Autodesk Fusion 360 part; units mm, degrees
(part 3 of 3)
  spline S39 degree 5 poles (-99.0173, 38.0348) (-99.0187, 38.0286) (-99.0216, 38.0164) (-99.0258, 37.9981) (-99.0314, 37.9737) (-99.0383, 37.9431) (-99.045, 37.9126) (-99.0515, 37.8821) (-99.058, 37.8516) (-99.0642, 37.8212) (-99.0704, 37.7907) (-99.0763, 37.7603) (-99.0822, 37.7298) (-99.0878, 37.6994) (-99.0934, 37.669) (-99.0987, 37.6387) (-99.104, 37.6083) (-99.1091, 37.578) (-99.114, 37.5477) (-99.1187, 37.5174) (-99.1234, 37.4871) (-99.1278, 37.4568) (-99.1321, 37.4266) (-99.1363, 37.3964) (-99.1403, 37.3662) (-99.1441, 37.3361) (-99.1478, 37.3059) (-99.1513, 37.2758) (-99.1546, 37.2457) (-99.1578, 37.2157) (-99.1608, 37.1857) (-99.1637, 37.1557) (-99.1663, 37.1257) (-99.1689, 37.0958) (-99.1712, 37.0659) (-99.1734, 37.036) (-99.1754, 37.0062) (-99.1772, 36.9764) (-99.1788, 36.9466) (-99.1803, 36.9169) (-99.1816, 36.8872) (-99.1827, 36.8576) (-99.1836, 36.8279) (-99.1843, 36.7984) (-99.1848, 36.7689) (-99.1851, 36.7394) (-99.1853, 36.7099) (-99.1852, 36.6805) (-99.185, 36.6512) (-99.1846, 36.6219) (-99.1839, 36.5926) (-99.183, 36.5634) (-99.1819, 36.5343) (-99.1805, 36.5052) (-99.179, 36.4762) (-99.1772, 36.4472) (-99.1752, 36.4183) (-99.173, 36.3895) (-99.1705, 36.3607) (-99.1679, 36.332) (-99.1649, 36.3033) (-99.1616, 36.2748) (-99.1579, 36.2463) (-99.1538, 36.218) (-99.1494, 36.1898) (-99.1448, 36.1616) (-99.1401, 36.1335) (-99.1351, 36.1054) (-99.1299, 36.0775) (-99.1242, 36.0497) (-99.1177, 36.0221) (-99.1117, 36.0003) (-99.1066, 35.9841) (-99.103, 35.9734) (-99.1011, 35.9681) knots -1 -1 -1 -1 -1 -1 -0.98571429 -0.97142857 -0.95714286 -0.94285714 -0.92857143 -0.91428571 -0.9 -0.88571429 -0.87142857 -0.85714286 -0.84285714 -0.82857143 -0.81428571 -0.8 -0.78571429 -0.77142857 -0.75714286 -0.74285714 -0.72857143 -0.71428571 -0.7 -0.68571429 -0.67142857 -0.65714286 -0.64285714 -0.62857143 -0.61428571 -0.6 -0.58571429 -0.57142857 -0.55714286 -0.54285714 -0.52857143 -0.51428571 -0.5 -0.48571429 -0.47142857 -0.45714286 -0.44285714 -0.42857143 -0.41428571 -0.4 -0.38571429 -0.37142857 -0.35714286 -0.34285714 -0.32857143 -0.31428571 -0.3 -0.28571429 -0.27142857 -0.25714286 -0.24285714 -0.22857143 -0.21428571 -0.2 -0.18571429 -0.17142857 -0.15714286 -0.14285714 -0.12857143 -0.11428571 -0.1 -0.08571429 -0.07142857 -0.05714286 -0.04285714 -0.02857143 -0.01428571 0 0 0 0 0 0
  line L39 (-99.1011, 35.9681) -> (-98.9382, 35.5089)
  arc A79 (-98.9981, 35.3816) -> (-98.9382, 35.5089) centre (-99.0325, 35.4755) ccw
  arc A80 (-98.9981, 35.3816) -> (-99.9434, 34.99) centre (-94.8448, 24.0176) ccw
  arc A81 (-100.0758, 35.0377) -> (-99.9434, 34.99) centre (-99.9856, 35.0807) ccw
  line L40 (-100.0758, 35.0377) -> (-100.2854, 35.4776)
  spline S40 degree 5 poles (-100.2854, 35.4776) (-100.2878, 35.4827) (-100.2928, 35.4928) (-100.3006, 35.5078) (-100.3118, 35.5275) (-100.3267, 35.5516) (-100.3423, 35.5753) (-100.3584, 35.5987) (-100.3747, 35.6221) (-100.3912, 35.6453) (-100.4079, 35.6685) (-100.4248, 35.6916) (-100.4419, 35.7145) (-100.4594, 35.7372) (-100.4773, 35.7597) (-100.4954, 35.7821) (-100.5138, 35.8043) (-100.5325, 35.8263) (-100.5513, 35.8483) (-100.5703, 35.8702) (-100.5896, 35.8919) (-100.609, 35.9135) (-100.6286, 35.9351) (-100.6484, 35.9565) (-100.6684, 35.9777) (-100.6886, 35.9989) (-100.709, 36.0199) (-100.7296, 36.0408) (-100.7504, 36.0617) (-100.7713, 36.0824) (-100.7924, 36.103) (-100.8136, 36.1235) (-100.835, 36.1439) (-100.8566, 36.1642) (-100.8783, 36.1844) (-100.9002, 36.2045) (-100.9223, 36.2245) (-100.9445, 36.2443) (-100.9669, 36.2641) (-100.9894, 36.2838) (-101.012, 36.3034) (-101.0348, 36.3229) (-101.0578, 36.3423) (-101.0808, 36.3616) (-101.1041, 36.3808) (-101.1274, 36.3999) (-101.1509, 36.4189) (-101.1746, 36.4378) (-101.1983, 36.4566) (-101.2222, 36.4753) (-101.2463, 36.4939) (-101.2704, 36.5124) (-101.2947, 36.5308) (-101.3191, 36.5492) (-101.3437, 36.5674) (-101.3683, 36.5855) (-101.3931, 36.6036) (-101.4181, 36.6215) (-101.4431, 36.6394) (-101.4683, 36.6572) (-101.4935, 36.6748) (-101.5189, 36.6924) (-101.5445, 36.7099) (-101.5701, 36.7273) (-101.5958, 36.7446) (-101.6217, 36.7618) (-101.6477, 36.7789) (-101.6738, 36.7959) (-101.7, 36.8129) (-101.7263, 36.8297) (-101.7527, 36.8465) (-101.774, 36.8598) (-101.7899, 36.8697) (-101.8006, 36.8763) (-101.806, 36.8797) knots 0 0 0 0 0 0 0.01428571 0.02857143 0.04285714 0.05714286 0.07142857 0.08571429 0.1 0.11428571 0.12857143 0.14285714 0.15714286 0.17142857 0.18571429 0.2 0.21428571 0.22857143 0.24285714 0.25714286 0.27142857 0.28571429 0.3 0.31428571 0.32857143 0.34285714 0.35714286 0.37142857 0.38571429 0.4 0.41428571 0.42857143 0.44285714 0.45714286 0.47142857 0.48571429 0.5 0.51428571 0.52857143 0.54285714 0.55714286 0.57142857 0.58571429 0.6 0.61428571 0.62857143 0.64285714 0.65714286 0.67142857 0.68571429 0.7 0.71428571 0.72857143 0.74285714 0.75714286 0.77142857 0.78571429 0.8 0.81428571 0.82857143 0.84285714 0.85714286 0.87142857 0.88571429 0.9 0.91428571 0.92857143 0.94285714 0.95714286 0.97142857 0.98571429 1 1 1 1 1 1
  arc A82 (-101.806, 36.8797) -> (-102.503, 36.4772) centre (-94.8448, 24.0176) ccw
  spline S41 degree 5 poles (-102.503, 36.4772) (-102.5028, 36.4709) (-102.5024, 36.4584) (-102.5018, 36.4396) (-102.5009, 36.4145) (-102.4996, 36.3833) (-102.4982, 36.3521) (-102.4966, 36.3209) (-102.4949, 36.2898) (-102.4931, 36.2587) (-102.4911, 36.2277) (-102.489, 36.1968) (-102.4868, 36.1659) (-102.4844, 36.135) (-102.4818, 36.1042) (-102.4792, 36.0735) (-102.4764, 36.0428) (-102.4734, 36.0122) (-102.4703, 35.9817) (-102.4671, 35.9512) (-102.4637, 35.9207) (-102.4602, 35.8904) (-102.4565, 35.86) (-102.4527, 35.8298) (-102.4488, 35.7996) (-102.4447, 35.7695) (-102.4404, 35.7394) (-102.436, 35.7095) (-102.4315, 35.6795) (-102.4268, 35.6497) (-102.4219, 35.6199) (-102.4169, 35.5902) (-102.4117, 35.5606) (-102.4064, 35.531) (-102.4009, 35.5015) (-102.3953, 35.4721) (-102.3895, 35.4428) (-102.3835, 35.4135) (-102.3774, 35.3843) (-102.3711, 35.3552) (-102.3647, 35.3262) (-102.3581, 35.2973) (-102.3513, 35.2685) (-102.3443, 35.2397) (-102.3372, 35.2111) (-102.3299, 35.1825) (-102.3224, 35.154) (-102.3148, 35.1256) (-102.3069, 35.0974) (-102.2989, 35.0692) (-102.2907, 35.0411) (-102.2823, 35.0131) (-102.2737, 34.9853) (-102.2648, 34.9575) (-102.2558, 34.9299) (-102.2466, 34.9024) (-102.2372, 34.875) (-102.2276, 34.8477) (-102.2178, 34.8205) (-102.2077, 34.7935) (-102.1975, 34.7666) (-102.1869, 34.7398) (-102.1759, 34.7133) (-102.1647, 34.687) (-102.1532, 34.6609) (-102.1414, 34.6349) (-102.1295, 34.6089) (-102.1175, 34.5831) (-102.1052, 34.5575) (-102.0925, 34.5321) (-102.0791, 34.5072) (-102.0676, 34.4877) (-102.0586, 34.4733) (-102.0523, 34.464) (-102.0491, 34.4593) knots -1 -1 -1 -1 -1 -1 -0.98571429 -0.97142857 -0.95714286 -0.94285714 -0.92857143 -0.91428571 -0.9 -0.88571429 -0.87142857 -0.85714286 -0.84285714 -0.82857143 -0.81428571 -0.8 -0.78571429 -0.77142857 -0.75714286 -0.74285714 -0.72857143 -0.71428571 -0.7 -0.68571429 -0.67142857 -0.65714286 -0.64285714 -0.62857143 -0.61428571 -0.6 -0.58571429 -0.57142857 -0.55714286 -0.54285714 -0.52857143 -0.51428571 -0.5 -0.48571429 -0.47142857 -0.45714286 -0.44285714 -0.42857143 -0.41428571 -0.4 -0.38571429 -0.37142857 -0.35714286 -0.34285714 -0.32857143 -0.31428571 -0.3 -0.28571429 -0.27142857 -0.25714286 -0.24285714 -0.22857143 -0.21428571 -0.2 -0.18571429 -0.17142857 -0.15714286 -0.14285714 -0.12857143 -0.11428571 -0.1 -0.08571429 -0.07142857 -0.05714286 -0.04285714 -0.02857143 -0.01428571 0 0 0 0 0 0
  line L41 (-102.0491, 34.4593) -> (-101.7729, 34.0579)
  arc A83 (-101.7978, 33.9194) -> (-101.7729, 34.0579) centre (-101.8553, 34.0012) ccw
  arc A84 (-101.7978, 33.9194) -> (-102.6096, 33.2965) centre (-94.8448, 24.0176) ccw
  arc A85 (-102.7498, 33.3083) -> (-102.6096, 33.2965) centre (-102.6737, 33.3732) ccw
  line L42 (-102.7498, 33.3083) -> (-103.066, 33.6789)
  spline S42 degree 5 poles (-103.066, 33.6789) (-103.0697, 33.6832) (-103.0772, 33.6917) (-103.0886, 33.7042) (-103.1045, 33.7203) (-103.1251, 33.7397) (-103.1464, 33.7586) (-103.168, 33.7771) (-103.1898, 33.7954) (-103.2117, 33.8136) (-103.2338, 33.8317) (-103.2561, 33.8496) (-103.2786, 33.8672) (-103.3014, 33.8847) (-103.3244, 33.9018) (-103.3477, 33.9187) (-103.3713, 33.9354) (-103.395, 33.9519) (-103.4189, 33.9682) (-103.4429, 33.9844) (-103.4671, 34.0004) (-103.4914, 34.0163) (-103.516, 34.032) (-103.5406, 34.0476) (-103.5655, 34.0629) (-103.5905, 34.0781) (-103.6156, 34.0932) (-103.6409, 34.108) (-103.6664, 34.1228) (-103.6919, 34.1374) (-103.7176, 34.1518) (-103.7435, 34.1661) (-103.7694, 34.1803) (-103.7955, 34.1943) (-103.8217, 34.2082) (-103.8481, 34.2219) (-103.8746, 34.2355) (-103.9012, 34.249) (-103.9279, 34.2623) (-103.9547, 34.2755) (-103.9817, 34.2886) (-104.0087, 34.3015) (-104.0359, 34.3143) (-104.0632, 34.3269) (-104.0906, 34.3395) (-104.1181, 34.3519) (-104.1457, 34.3641) (-104.1734, 34.3763) (-104.2013, 34.3883) (-104.2292, 34.4002) (-104.2572, 34.4119) (-104.2854, 34.4236) (-104.3136, 34.4351) (-104.3419, 34.4465) (-104.3704, 34.4577) (-104.3989, 34.4689) (-104.4275, 34.4799) (-104.4562, 34.4908) (-104.485, 34.5015) (-104.5139, 34.5122) (-104.5429, 34.5227) (-104.572, 34.5331) (-104.6012, 34.5434) (-104.6304, 34.5536) (-104.6598, 34.5636) (-104.6892, 34.5736) (-104.7188, 34.5834) (-104.7484, 34.5931) (-104.7781, 34.6026) (-104.8078, 34.6121) (-104.8377, 34.6214) (-104.8617, 34.6288) (-104.8797, 34.6343) (-104.8917, 34.6379) (-104.8977, 34.6397) knots 0 0 0 0 0 0 0.01428571 0.02857143 0.04285714 0.05714286 0.07142857 0.08571429 0.1 0.11428571 0.12857143 0.14285714 0.15714286 0.17142857 0.18571429 0.2 0.21428571 0.22857143 0.24285714 0.25714286 0.27142857 0.28571429 0.3 0.31428571 0.32857143 0.34285714 0.35714286 0.37142857 0.38571429 0.4 0.41428571 0.42857143 0.44285714 0.45714286 0.47142857 0.48571429 0.5 0.51428571 0.52857143 0.54285714 0.55714286 0.57142857 0.58571429 0.6 0.61428571 0.62857143 0.64285714 0.65714286 0.67142857 0.68571429 0.7 0.71428571 0.72857143 0.74285714 0.75714286 0.77142857 0.78571429 0.8 0.81428571 0.82857143 0.84285714 0.85714286 0.87142857 0.88571429 0.9 0.91428571 0.92857143 0.94285714 0.95714286 0.97142857 0.98571429 1 1 1 1 1 1
  arc A86 (-104.8977, 34.6397) -> (-105.4668, 34.0706) centre (-94.8448, 24.0176) ccw
  spline S43 degree 5 poles (-105.4668, 34.0706) (-105.465, 34.0645) (-105.4614, 34.0525) (-105.4559, 34.0345) (-105.4486, 34.0106) (-105.4392, 33.9807) (-105.4298, 33.9509) (-105.4202, 33.9212) (-105.4105, 33.8916) (-105.4007, 33.8621) (-105.3908, 33.8327) (-105.3807, 33.8033) (-105.3706, 33.774) (-105.3603, 33.7449) (-105.3499, 33.7158) (-105.3393, 33.6868) (-105.3287, 33.6579) (-105.3179, 33.6291) (-105.307, 33.6004) (-105.296, 33.5717) (-105.2849, 33.5432) (-105.2736, 33.5148) (-105.2622, 33.4865) (-105.2507, 33.4582) (-105.2391, 33.4301) (-105.2273, 33.4021) (-105.2154, 33.3741) (-105.2034, 33.3463) (-105.1913, 33.3186) (-105.179, 33.291) (-105.1666, 33.2635) (-105.1541, 33.2361) (-105.1414, 33.2088) (-105.1286, 33.1816) (-105.1157, 33.1545) (-105.1027, 33.1276) (-105.0895, 33.1007) (-105.0761, 33.074) (-105.0627, 33.0474) (-105.0491, 33.021) (-105.0353, 32.9946) (-105.0215, 32.9684) (-105.0075, 32.9423) (-104.9933, 32.9163) (-104.979, 32.8905) (-104.9645, 32.8648) (-104.9499, 32.8392) (-104.9352, 32.8138) (-104.9203, 32.7885) (-104.9053, 32.7633) (-104.8901, 32.7383) (-104.8747, 32.7135) (-104.8592, 32.6888) (-104.8435, 32.6643) (-104.8276, 32.64) (-104.8116, 32.6158) (-104.7954, 32.5917) (-104.779, 32.5679) (-104.7625, 32.5441) (-104.7459, 32.5206) (-104.729, 32.4973) (-104.7118, 32.4742) (-104.6944, 32.4514) (-104.6767, 32.4289) (-104.6588, 32.4067) (-104.6407, 32.3846) (-104.6225, 32.3626) (-104.6042, 32.3408) (-104.5857, 32.3192) (-104.5669, 32.298) (-104.5475, 32.2774) (-104.5314, 32.2615) (-104.5189, 32.25) (-104.5104, 32.2426) (-104.5061, 32.2389) knots -1 -1 -1 -1 -1 -1 -0.98571429 -0.97142857 -0.95714286 -0.94285714 -0.92857143 -0.91428571 -0.9 -0.88571429 -0.87142857 -0.85714286 -0.84285714 -0.82857143 -0.81428571 -0.8 -0.78571429 -0.77142857 -0.75714286 -0.74285714 -0.72857143 -0.71428571 -0.7 -0.68571429 -0.67142857 -0.65714286 -0.64285714 -0.62857143 -0.61428571 -0.6 -0.58571429 -0.57142857 -0.55714286 -0.54285714 -0.52857143 -0.51428571 -0.5 -0.48571429 -0.47142857 -0.45714286 -0.44285714 -0.42857143 -0.41428571 -0.4 -0.38571429 -0.37142857 -0.35714286 -0.34285714 -0.32857143 -0.31428571 -0.3 -0.28571429 -0.27142857 -0.25714286 -0.24285714 -0.22857143 -0.21428571 -0.2 -0.18571429 -0.17142857 -0.15714286 -0.14285714 -0.12857143 -0.11428571 -0.1 -0.08571429 -0.07142857 -0.05714286 -0.04285714 -0.02857143 -0.01428571 0 0 0 0 0 0
  line L43 (-104.5061, 32.2389) -> (-104.1355, 31.9227)
  arc A87 (-104.1237, 31.7824) -> (-104.1355, 31.9227) centre (-104.2004, 31.8466) ccw
  arc A88 (-104.1237, 31.7824) -> (-104.7465, 30.9707) centre (-94.8448, 24.0176) ccw
  arc A89 (-104.8851, 30.9458) -> (-104.7465, 30.9707) centre (-104.8284, 31.0281) ccw
  line L44 (-104.8851, 30.9458) -> (-105.2864, 31.2219)
  spline S44 degree 5 poles (-105.2864, 31.2219) (-105.2911, 31.2251) (-105.3005, 31.2314) (-105.3148, 31.2405) (-105.3343, 31.2519) (-105.3593, 31.2653) (-105.3846, 31.278) (-105.4103, 31.2903) (-105.4361, 31.3024) (-105.462, 31.3143) (-105.488, 31.326) (-105.5142, 31.3375) (-105.5405, 31.3488) (-105.567, 31.3597) (-105.5937, 31.3703) (-105.6206, 31.3806) (-105.6477, 31.3906) (-105.6748, 31.4004) (-105.7021, 31.41) (-105.7295, 31.4194) (-105.7571, 31.4287) (-105.7847, 31.4377) (-105.8124, 31.4465) (-105.8403, 31.4551) (-105.8682, 31.4636) (-105.8963, 31.4718) (-105.9245, 31.4798) (-105.9528, 31.4876) (-105.9812, 31.4953) (-106.0097, 31.5027) (-106.0382, 31.51) (-106.0669, 31.5172) (-106.0956, 31.5241) (-106.1245, 31.5309) (-106.1534, 31.5375) (-106.1824, 31.544) (-106.2115, 31.5503) (-106.2407, 31.5564) (-106.2699, 31.5623) (-106.2993, 31.5681) (-106.3287, 31.5738) (-106.3581, 31.5793) (-106.3877, 31.5846) (-106.4173, 31.5897) (-106.4471, 31.5948) (-106.4768, 31.5996) (-106.5067, 31.6043) (-106.5366, 31.6089) (-106.5666, 31.6133) (-106.5966, 31.6175) (-106.6268, 31.6216) (-106.6569, 31.6256) (-106.6872, 31.6294) (-106.7175, 31.6331) (-106.7479, 31.6366) (-106.7783, 31.64) (-106.8088, 31.6432) (-106.8394, 31.6463) (-106.87, 31.6492) (-106.9007, 31.652) (-106.9314, 31.6547) (-106.9622, 31.6572) (-106.993, 31.6596) (-107.0239, 31.6619) (-107.0549, 31.664) (-107.0859, 31.6659) (-107.1169, 31.6678) (-107.148, 31.6695) (-107.1792, 31.671) (-107.2104, 31.6724) (-107.2417, 31.6737) (-107.2667, 31.6746) (-107.2855, 31.6753) (-107.2981, 31.6757) (-107.3044, 31.6759) knots 0 0 0 0 0 0 0.01428571 0.02857143 0.04285714 0.05714286 0.07142857 0.08571429 0.1 0.11428571 0.12857143 0.14285714 0.15714286 0.17142857 0.18571429 0.2 0.21428571 0.22857143 0.24285714 0.25714286 0.27142857 0.28571429 0.3 0.31428571 0.32857143 0.34285714 0.35714286 0.37142857 0.38571429 0.4 0.41428571 0.42857143 0.44285714 0.45714286 0.47142857 0.48571429 0.5 0.51428571 0.52857143 0.54285714 0.55714286 0.57142857 0.58571429 0.6 0.61428571 0.62857143 0.64285714 0.65714286 0.67142857 0.68571429 0.7 0.71428571 0.72857143 0.74285714 0.75714286 0.77142857 0.78571429 0.8 0.81428571 0.82857143 0.84285714 0.85714286 0.87142857 0.88571429 0.9 0.91428571 0.92857143 0.94285714 0.95714286 0.97142857 0.98571429 1 1 1 1 1 1
  arc A90 (-107.3044, 31.6759) -> (-107.7068, 30.9788) centre (-94.8448, 24.0176) ccw
  spline S45 degree 5 poles (-107.7068, 30.9788) (-107.7035, 30.9735) (-107.6969, 30.9628) (-107.6869, 30.9468) (-107.6736, 30.9256) (-107.6569, 30.8992) (-107.64, 30.8728) (-107.6231, 30.8466) (-107.6061, 30.8205) (-107.589, 30.7946) (-107.5718, 30.7687) (-107.5544, 30.7429) (-107.5371, 30.7173) (-107.5196, 30.6918) (-107.502, 30.6664) (-107.4843, 30.6411) (-107.4666, 30.616) (-107.4487, 30.5909) (-107.4307, 30.566) (-107.4127, 30.5412) (-107.3945, 30.5165) (-107.3763, 30.492) (-107.358, 30.4676) (-107.3396, 30.4433) (-107.321, 30.4191) (-107.3024, 30.3951) (-107.2837, 30.3712) (-107.2649, 30.3474) (-107.246, 30.3238) (-107.227, 30.3003) (-107.2079, 30.2769) (-107.1887, 30.2537) (-107.1694, 30.2306) (-107.15, 30.2077) (-107.1305, 30.1849) (-107.111, 30.1622) (-107.0913, 30.1397) (-107.0715, 30.1174) (-107.0516, 30.0952) (-107.0316, 30.0731) (-107.0115, 30.0512) (-106.9913, 30.0295) (-106.971, 30.0079) (-106.9506, 29.9865) (-106.9301, 29.9652) (-106.9095, 29.9441) (-106.8888, 29.9232) (-106.868, 29.9025) (-106.8471, 29.8819) (-106.826, 29.8615) (-106.8049, 29.8412) (-106.7836, 29.8212) (-106.7622, 29.8014) (-106.7407, 29.7818) (-106.7191, 29.7624) (-106.6973, 29.7432) (-106.6755, 29.7242) (-106.6535, 29.7053) (-106.6314, 29.6867) (-106.6092, 29.6683) (-106.5869, 29.6501) (-106.5643, 29.6323) (-106.5416, 29.6148) (-106.5187, 29.5976) (-106.4956, 29.5807) (-106.4725, 29.5641) (-106.4492, 29.5476) (-106.4259, 29.5313) (-106.4024, 29.5152) (-106.3787, 29.4996) (-106.3546, 29.4847) (-106.335, 29.4735) (-106.32, 29.4656) (-106.3098, 29.4607) (-106.3047, 29.4582) knots -1 -1 -1 -1 -1 -1 -0.98571429 -0.97142857 -0.95714286 -0.94285714 -0.92857143 -0.91428571 -0.9 -0.88571429 -0.87142857 -0.85714286 -0.84285714 -0.82857143 -0.81428571 -0.8 -0.78571429 -0.77142857 -0.75714286 -0.74285714 -0.72857143 -0.71428571 -0.7 -0.68571429 -0.67142857 -0.65714286 -0.64285714 -0.62857143 -0.61428571 -0.6 -0.58571429 -0.57142857 -0.55714286 -0.54285714 -0.52857143 -0.51428571 -0.5 -0.48571429 -0.47142857 -0.45714286 -0.44285714 -0.42857143 -0.41428571 -0.4 -0.38571429 -0.37142857 -0.35714286 -0.34285714 -0.32857143 -0.31428571 -0.3 -0.28571429 -0.27142857 -0.25714286 -0.24285714 -0.22857143 -0.21428571 -0.2 -0.18571429 -0.17142857 -0.15714286 -0.14285714 -0.12857143 -0.11428571 -0.1 -0.08571429 -0.07142857 -0.05714286 -0.04285714 -0.02857143 -0.01428571 0 0 0 0 0 0
  line L45 (-106.3047, 29.4582) -> (-105.8649, 29.2487)
  arc A91 (-105.8172, 29.1163) -> (-105.8649, 29.2487) centre (-105.9079, 29.1584) ccw
  arc A92 (-105.8172, 29.1163) -> (-106.2087, 28.171) centre (-94.8448, 24.0176) ccw
  arc A93 (-106.3361, 28.1111) -> (-106.2087, 28.171) centre (-106.3027, 28.2053) ccw
  line L46 (-106.3361, 28.1111) -> (-106.7953, 28.2739)
  spline S46 degree 5 poles (-106.7953, 28.2739) (-106.8006, 28.2758) (-106.8113, 28.2795) (-106.8275, 28.2845) (-106.8493, 28.2905) (-106.8768, 28.297) (-106.9046, 28.3027) (-106.9326, 28.3079) (-106.9606, 28.3129) (-106.9887, 28.3177) (-107.0169, 28.3223) (-107.0452, 28.3267) (-107.0735, 28.3307) (-107.1019, 28.3344) (-107.1305, 28.3377) (-107.1591, 28.3407) (-107.1878, 28.3434) (-107.2166, 28.3458) (-107.2455, 28.348) (-107.2744, 28.35) (-107.3033, 28.3518) (-107.3324, 28.3534) (-107.3614, 28.3547) (-107.3906, 28.3559) (-107.4198, 28.3567) (-107.449, 28.3574) (-107.4783, 28.3579) (-107.5077, 28.3581) (-107.5371, 28.3581) (-107.5665, 28.358) (-107.596, 28.3577) (-107.6255, 28.3571) (-107.6551, 28.3564) (-107.6847, 28.3555) (-107.7144, 28.3544) (-107.744, 28.3531) (-107.7738, 28.3517) (-107.8035, 28.35) (-107.8333, 28.3482) (-107.8632, 28.3462) (-107.893, 28.3441) (-107.9229, 28.3417) (-107.9529, 28.3392) (-107.9828, 28.3365) (-108.0128, 28.3337) (-108.0428, 28.3307) (-108.0729, 28.3275) (-108.103, 28.3241) (-108.1331, 28.3206) (-108.1632, 28.3169) (-108.1934, 28.3131) (-108.2235, 28.3091) (-108.2538, 28.305) (-108.284, 28.3007) (-108.3142, 28.2962) (-108.3445, 28.2916) (-108.3748, 28.2868) (-108.4051, 28.2819) (-108.4354, 28.2768) (-108.4658, 28.2716) (-108.4962, 28.2662) (-108.5266, 28.2607) (-108.557, 28.255) (-108.5874, 28.2492) (-108.6178, 28.2432) (-108.6483, 28.2371) (-108.6788, 28.2308) (-108.7093, 28.2244) (-108.7398, 28.2178) (-108.7703, 28.2111) (-108.8008, 28.2043) (-108.8252, 28.1987) (-108.8436, 28.1944) (-108.8558, 28.1916) (-108.8619, 28.1901) knots 0 0 0 0 0 0 0.01428571 0.02857143 0.04285714 0.05714286 0.07142857 0.08571429 0.1 0.11428571 0.12857143 0.14285714 0.15714286 0.17142857 0.18571429 0.2 0.21428571 0.22857143 0.24285714 0.25714286 0.27142857 0.28571429 0.3 0.31428571 0.32857143 0.34285714 0.35714286 0.37142857 0.38571429 0.4 0.41428571 0.42857143 0.44285714 0.45714286 0.47142857 0.48571429 0.5 0.51428571 0.52857143 0.54285714 0.55714286 0.57142857 0.58571429 0.6 0.61428571 0.62857143 0.64285714 0.65714286 0.67142857 0.68571429 0.7 0.71428571 0.72857143 0.74285714 0.75714286 0.77142857 0.78571429 0.8 0.81428571 0.82857143 0.84285714 0.85714286 0.87142857 0.88571429 0.9 0.91428571 0.92857143 0.94285714 0.95714286 0.97142857 0.98571429 1 1 1 1 1 1
  arc A94 (-108.8619, 28.1901) -> (-109.0702, 27.4127) centre (-94.8448, 24.0176) ccw
  spline S47 degree 5 poles (-109.0702, 27.4127) (-109.0657, 27.4084) (-109.0565, 27.3998) (-109.0428, 27.3869) (-109.0244, 27.3699) (-109.0014, 27.3487) (-108.9783, 27.3276) (-108.9552, 27.3067) (-108.932, 27.2859) (-108.9087, 27.2652) (-108.8854, 27.2447) (-108.862, 27.2243) (-108.8386, 27.204) (-108.8151, 27.1839) (-108.7915, 27.1639) (-108.7679, 27.1441) (-108.7443, 27.1244) (-108.7205, 27.1048) (-108.6967, 27.0854) (-108.6729, 27.0661) (-108.649, 27.047) (-108.625, 27.028) (-108.601, 27.0091) (-108.5769, 26.9904) (-108.5527, 26.9719) (-108.5285, 26.9535) (-108.5043, 26.9352) (-108.48, 26.9172) (-108.4556, 26.8992) (-108.4312, 26.8814) (-108.4067, 26.8638) (-108.3821, 26.8464) (-108.3575, 26.829) (-108.3328, 26.8119) (-108.3081, 26.7949) (-108.2833, 26.7781) (-108.2585, 26.7615) (-108.2336, 26.745) (-108.2086, 26.7287) (-108.1836, 26.7126) (-108.1586, 26.6966) (-108.1334, 26.6808) (-108.1082, 26.6652) (-108.083, 26.6498) (-108.0577, 26.6346) (-108.0323, 26.6196) (-108.0069, 26.6047) (-107.9814, 26.5901) (-107.9559, 26.5756) (-107.9303, 26.5614) (-107.9046, 26.5473) (-107.8789, 26.5335) (-107.8531, 26.5199) (-107.8272, 26.5065) (-107.8013, 26.4934) (-107.7753, 26.4804) (-107.7493, 26.4677) (-107.7232, 26.4552) (-107.6971, 26.4429) (-107.6709, 26.4309) (-107.6446, 26.4191) (-107.6182, 26.4077) (-107.5917, 26.3967) (-107.5651, 26.386) (-107.5385, 26.3757) (-107.5118, 26.3656) (-107.4851, 26.3557) (-107.4583, 26.346) (-107.4315, 26.3365) (-107.4045, 26.3276) (-107.3774, 26.3194) (-107.3556, 26.3137) (-107.339, 26.31) (-107.3279, 26.3078) (-107.3224, 26.3068) knots -1 -1 -1 -1 -1 -1 -0.98571429 -0.97142857 -0.95714286 -0.94285714 -0.92857143 -0.91428571 -0.9 -0.88571429 -0.87142857 -0.85714286 -0.84285714 -0.82857143 -0.81428571 -0.8 -0.78571429 -0.77142857 -0.75714286 -0.74285714 -0.72857143 -0.71428571 -0.7 -0.68571429 -0.67142857 -0.65714286 -0.64285714 -0.62857143 -0.61428571 -0.6 -0.58571429 -0.57142857 -0.55714286 -0.54285714 -0.52857143 -0.51428571 -0.5 -0.48571429 -0.47142857 -0.45714286 -0.44285714 -0.42857143 -0.41428571 -0.4 -0.38571429 -0.37142857 -0.35714286 -0.34285714 -0.32857143 -0.31428571 -0.3 -0.28571429 -0.27142857 -0.25714286 -0.24285714 -0.22857143 -0.21428571 -0.2 -0.18571429 -0.17142857 -0.15714286 -0.14285714 -0.12857143 -0.11428571 -0.1 -0.08571429 -0.07142857 -0.05714286 -0.04285714 -0.02857143 -0.01428571 0 0 0 0 0 0
  line L47 (-107.3224, 26.3068) -> (-106.8433, 26.2182)
  arc A95 (-106.7629, 26.1027) -> (-106.8433, 26.2182) centre (-106.8614, 26.1199) ccw
  circle A96 centre (-94.8448, 24.0176) radius 1.5
  line L48 (-94.8448, 26.5176) -> (-125.8448, 26.5176)
  arc A97 (-125.8448, 26.5176) -> (-125.8448, 21.5176) centre (-125.8448, 24.0176) ccw
  line L49 (-125.8448, 21.5176) -> (-94.8448, 21.5176)
  arc A98 (-94.8448, 21.5176) -> (-94.8448, 26.5176) centre (-94.8448, 24.0176) ccw
  line L50 (-94.8448, 24.0176) -> (-125.8448, 24.0176) construction
  circle A99 centre (-125.8448, 24.0176) radius 1.5
  dimension "d1" = 31
  dimension "d2" = 5
  dimension "d3" = 3
  constraint tangent L48 A97
  constraint tangent A97 L49
  constraint parallel L48 L49
  constraint tangent L49 A98
  constraint tangent L48 A98
  constraint horizontal L50
  constraint coincident A0.centre A2.centre
  constraint concentric A97 A99
  measures "d1" distance of A0.centre A97.centre
  measures "d2" diameter of A97
  measures "d3" diameter of A99
sketch "Sketch1" plane through (0, 0, 0) normal (0, 0, 1) x (1, 0, 0)
  circle A0 centre (0, 0) radius 12.0992
  circle A1 centre (0, 0) radius 1.5
  measures "d1" distance of A0.centre
sketch "Sketch2" plane through (0, 0, 0) normal (0, 0, 1) x (1, 0, 0)
  spline S0 degree 5 poles (12.6449, -1.0183) (12.6506, -1.0187) (12.6618, -1.0195) (12.6788, -1.0202) (12.7014, -1.0203) (12.7297, -1.0195) (12.758, -1.0178) (12.7864, -1.0156) (12.8147, -1.0131) (12.8431, -1.0105) (12.8715, -1.0076) (12.8999, -1.0045) (12.9284, -1.0011) (12.9568, -0.9973) (12.9852, -0.9932) (13.0137, -0.9886) (13.0421, -0.9838) (13.0705, -0.9787) (13.099, -0.9733) (13.1274, -0.9678) (13.1559, -0.962) (13.1843, -0.956) (13.2127, -0.9498) (13.2412, -0.9433) (13.2696, -0.9366) (13.298, -0.9297) (13.3264, -0.9226) (13.3549, -0.9152) (13.3833, -0.9076) (13.4117, -0.8999) (13.4401, -0.8919) (13.4684, -0.8838) (13.4968, -0.8754) (13.5252, -0.8669) (13.5535, -0.8581) (13.5819, -0.8492) (13.6102, -0.8401) (13.6385, -0.8308) (13.6669, -0.8214) (13.6952, -0.8117) (13.7234, -0.8019) (13.7517, -0.7919) (13.78, -0.7817) (13.8082, -0.7714) (13.8365, -0.7609) (13.8647, -0.7502) (13.8929, -0.7393) (13.9211, -0.7283) (13.9492, -0.7171) (13.9774, -0.7058) (14.0055, -0.6943) (14.0337, -0.6826) (14.0618, -0.6708) (14.0898, -0.6588) (14.1179, -0.6467) (14.146, -0.6344) (14.174, -0.6219) (14.202, -0.6093) (14.23, -0.5966) (14.2579, -0.5837) (14.2859, -0.5706) (14.3138, -0.5574) (14.3417, -0.544) (14.3696, -0.5305) (14.3975, -0.5169) (14.4253, -0.5031) (14.4531, -0.4891) (14.4809, -0.4751) (14.5087, -0.4608) (14.5364, -0.4465) (14.5641, -0.4319) (14.5863, -0.4202) (14.6029, -0.4114) (14.6139, -0.4054) (14.6195, -0.4024) knots 0 0 0 0 0 0 0.01428571 0.02857143 0.04285714 0.05714286 0.07142857 0.08571429 0.1 0.11428571 0.12857143 0.14285714 0.15714286 0.17142857 0.18571429 0.2 0.21428571 0.22857143 0.24285714 0.25714286 0.27142857 0.28571429 0.3 0.31428571 0.32857143 0.34285714 0.35714286 0.37142857 0.38571429 0.4 0.41428571 0.42857143 0.44285714 0.45714286 0.47142857 0.48571429 0.5 0.51428571 0.52857143 0.54285714 0.55714286 0.57142857 0.58571429 0.6 0.61428571 0.62857143 0.64285714 0.65714286 0.67142857 0.68571429 0.7 0.71428571 0.72857143 0.74285714 0.75714286 0.77142857 0.78571429 0.8 0.81428571 0.82857143 0.84285714 0.85714286 0.87142857 0.88571429 0.9 0.91428571 0.92857143 0.94285714 0.95714286 0.97142857 0.98571429 1 1 1 1 1 1
  spline S1 degree 5 poles (12.6449, 1.0183) (12.6506, 1.0187) (12.6618, 1.0195) (12.6788, 1.0202) (12.7014, 1.0203) (12.7297, 1.0195) (12.758, 1.0178) (12.7864, 1.0156) (12.8147, 1.0131) (12.8431, 1.0105) (12.8715, 1.0076) (12.8999, 1.0045) (12.9284, 1.0011) (12.9568, 0.9973) (12.9852, 0.9932) (13.0137, 0.9886) (13.0421, 0.9838) (13.0705, 0.9787) (13.099, 0.9733) (13.1274, 0.9678) (13.1559, 0.962) (13.1843, 0.956) (13.2127, 0.9498) (13.2412, 0.9433) (13.2696, 0.9366) (13.298, 0.9297) (13.3264, 0.9226) (13.3549, 0.9152) (13.3833, 0.9076) (13.4117, 0.8999) (13.4401, 0.8919) (13.4684, 0.8838) (13.4968, 0.8754) (13.5252, 0.8669) (13.5535, 0.8581) (13.5819, 0.8492) (13.6102, 0.8401) (13.6385, 0.8308) (13.6669, 0.8214) (13.6952, 0.8117) (13.7234, 0.8019) (13.7517, 0.7919) (13.78, 0.7817) (13.8082, 0.7714) (13.8365, 0.7609) (13.8647, 0.7502) (13.8929, 0.7393) (13.9211, 0.7283) (13.9492, 0.7171) (13.9774, 0.7058) (14.0055, 0.6943) (14.0337, 0.6826) (14.0618, 0.6708) (14.0898, 0.6588) (14.1179, 0.6467) (14.146, 0.6344) (14.174, 0.6219) (14.202, 0.6093) (14.23, 0.5966) (14.2579, 0.5837) (14.2859, 0.5706) (14.3138, 0.5574) (14.3417, 0.544) (14.3696, 0.5305) (14.3975, 0.5169) (14.4253, 0.5031) (14.4531, 0.4891) (14.4809, 0.4751) (14.5087, 0.4608) (14.5364, 0.4465) (14.5641, 0.4319) (14.5863, 0.4202) (14.6029, 0.4114) (14.6139, 0.4054) (14.6195, 0.4024) knots 0 0 0 0 0 0 0.01428571 0.02857143 0.04285714 0.05714286 0.07142857 0.08571429 0.1 0.11428571 0.12857143 0.14285714 0.15714286 0.17142857 0.18571429 0.2 0.21428571 0.22857143 0.24285714 0.25714286 0.27142857 0.28571429 0.3 0.31428571 0.32857143 0.34285714 0.35714286 0.37142857 0.38571429 0.4 0.41428571 0.42857143 0.44285714 0.45714286 0.47142857 0.48571429 0.5 0.51428571 0.52857143 0.54285714 0.55714286 0.57142857 0.58571429 0.6 0.61428571 0.62857143 0.64285714 0.65714286 0.67142857 0.68571429 0.7 0.71428571 0.72857143 0.74285714 0.75714286 0.77142857 0.78571429 0.8 0.81428571 0.82857143 0.84285714 0.85714286 0.87142857 0.88571429 0.9 0.91428571 0.92857143 0.94285714 0.95714286 0.97142857 0.98571429 1 1 1 1 1 1
  arc A0 (14.6195, -0.4024) -> (14.6195, 0.4024) centre (0, 0) ccw
  line L0 (12.0502, -0.9712) -> (12.6449, -1.0183)
  line L1 (12.0502, 0.9712) -> (12.6449, 1.0183)
  line L2 (12.0502, -0.9712) -> (12.0502, 0.9712)
  point P0 (12.7841, -1.0157)
  point P1 (12.9241, -1.0016)
  point P2 (13.0647, -0.9797)
  point P3 (13.2057, -0.9513)
  point P4 (13.3469, -0.9172)
  point P5 (13.4884, -0.8779)
  point P6 (13.63, -0.8336)
  point P7 (13.7716, -0.7847)
  point P8 (13.9132, -0.7313)
  point P9 (14.0548, -0.6737)
  point P10 (14.1963, -0.6119)
  point P11 (14.3376, -0.546)
  point P12 (14.4787, -0.4761)
  point P13 (12.7841, 1.0157)
  point P14 (12.9241, 1.0016)
  point P15 (13.0647, 0.9797)
  point P16 (13.2057, 0.9513)
  point P17 (13.3469, 0.9172)
  point P18 (13.4884, 0.8779)
  point P19 (13.63, 0.8336)
  point P20 (13.7716, 0.7847)
  point P21 (13.9132, 0.7313)
  point P22 (14.0548, 0.6737)
  point P23 (14.1963, 0.6119)
  point P24 (14.3376, 0.546)
  point P25 (14.4787, 0.4761)
sketch "Sketch3" plane through (0, 0, 0) normal (0, 0, 1) x (1, 0, 0)
  circle A0 centre (0, 0) radius 13.5 construction
extrude "Extrude3" add sketch "Sketch4" against normal blind 5
move_body "Move1" bodies 1 to x (1, 0, 0) y (0, 1, 0) z (0, 0, 1) at (-25, -15, -65)
